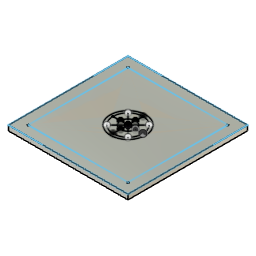
Rotator_Base_Mount_v9 (Autodesk Fusion 360 design; units mm, degrees)
Autodesk Fusion 360 part; units mm, degrees
sketch "Sketch1" plane through (0, 0, 0) normal (0, 0, 1) x (1, 0, 0)
  line L0 (-152.4, -152.4) -> (152.4, -152.4)
  line L1 (152.4, -152.4) -> (152.4, 152.4)
  line L2 (152.4, 152.4) -> (-152.4, 152.4)
  line L3 (-152.4, 152.4) -> (-152.4, -152.4)
  line L4 (-127, -127) -> (127, -127)
  line L5 (127, -127) -> (127, 127)
  line L6 (127, 127) -> (-127, 127)
  line L7 (-127, 127) -> (-127, -127)
  circle A0 centre (0, 0) radius 45
  circle A1 centre (0, 0) radius 38.1
  circle A2 centre (0, 0) radius 19.05
  line L8 (0, 0) -> (-38.1, 0)
  line L9 (0, 0) -> (0, 38.1)
  line L10 (0, 0) -> (38.1, 0)
  line L11 (0, 0) -> (0, -38.1)
  line L12 (0, 0) -> (26.9408, 26.9408)
  line L13 (0, 0) -> (38.1, 0) construction
  line L14 (0, 0) -> (26.9408, -26.9408)
  line L15 (0, 0) -> (38.1, 0) construction
  line L16 (0, 0) -> (-26.9408, -26.9408)
  line L17 (0, 0) -> (38.1, 0) construction
  line L18 (0, 0) -> (-26.9408, 26.9408)
  line L19 (0, 0) -> (38.1, 0) construction
  point P0 (0, 19.05)
  point P1 (19.05, 0)
  point P2 (0, -19.05)
  point P3 (-19.05, 0)
  dimension "d1" = 304.8
  dimension "d2" = 304.8
  dimension "d3" = 254
  dimension "d4" = 254
  dimension "d5" = 90
  dimension "d6" = 76.2
  dimension "d7" = 38.1
  dimension "d8" = 38.1
  dimension "d9" = 38.1
  dimension "d10" = 38.1
  dimension "d11" = 38.1
  dimension "d12" = 45
  dimension "d13" = 45
  dimension "d14" = 135
  dimension "d15" = 135
  constraint horizontal L0
  constraint vertical L1
  constraint horizontal L2
  constraint vertical L3
  constraint horizontal L4
  constraint vertical L5
  constraint horizontal L6
  constraint vertical L7
  constraint coincident A0.centre A1.centre
  constraint coincident A1 L8.end
  constraint horizontal L8
  constraint perpendicular L8 L9
  constraint parallel L8 L10
  constraint perpendicular L10 L11
  constraint horizontal L13
  constraint horizontal L15
  constraint horizontal L17
  constraint horizontal L19
  constraint midpoint L9 P0
  constraint midpoint L17 P1
  constraint midpoint L11 P2
  constraint midpoint L8 P3
  measures "d1" distance of L0.start L0.end
  measures "d2" distance of L0.start L2.end
  measures "d3" distance of L4.start L4.end
  measures "d4" distance of L4.start L6.end
  measures "d5" diameter of A0
  measures "d6" diameter of A1
  measures "d7" diameter of A2
  measures "d8" distance of A0.centre L8.end
  measures "d9" distance of A0.centre L9.end
  measures "d10" distance of A0.centre L10.end
  measures "d11" distance of A0.centre L11.end
  measures "d12" angle of L12 L13
  measures "d13" angle of L14 L15
  measures "d14" angle of L16 L17
  measures "d15" angle of L18 L19
extrude "Extrude1" add sketch "Sketch1" against normal blind 12.7 contours L0 L1 L2 L3 | L4 L5 L6 L7 | A0 | A1 A2 L10 L12 | A1 A2 L10 L14 | A1 A2 L9 L12 | A1 A2 L11 L14 | A2 L10 L12 | A2 L10 L14 | A1 A2 L9 L18 | A2 L9 L12 | A1 A2 L11 L16 | A2 L11 L14 | A2 L8 L16 | A2 L9 L18 | A2 L11 L16 | A2 L8 L18 | A1 A2 L8 L18 | A1 A2 L8 L16 makes body 1 in component "PT785S_Base_Mount"
hole "Hole1" at (-127, 127, 0) at (127, 127, 0) at (127, -127, 0) at (-127, -127, 0) at (-38.1, 0, 0) at (0, 38.1, 0) at (38.1, 0, 0) at (0, -38.1, 0) direction (0, 0, -1) diameter 5.1308 depth 12.7 tip angle 180 bodies 1 in component "PT785S_Base_Mount"
thread "Thread1" "ANSI Unified Screw Threads 0.25 1/4-20 UNC 1B" in component "PT785S_Base_Mount"
hole "Hole2" at (-26.9408, 26.9408, 0) at (26.9408, 26.9408, 0) at (26.9408, -26.9408, 0) at (-26.9408, -26.9408, 0) at (-19.05, 0, 0) at (0, 19.05, 0) at (19.05, 0, 0) at (0, -19.05, 0) direction (0, 0, -1) diameter 2.7686 depth 12.7 tip angle 180 bodies 1 in component "PT785S_Base_Mount"
thread "Thread2" "ANSI Unified Screw Threads 0.138(#6) 6-32 UNC 2B" in component "PT785S_Base_Mount"
hole "Hole3" at (0, 0, 0) direction (0, 0, -1) diameter 7.9756 depth 12.7 tip angle 180 bodies 1 in component "PT785S_Base_Mount"
thread "Thread3" "ANSI Unified Screw Threads 0.375 3/8-16 UNC 1B" in component "PT785S_Base_Mount"
copy_body "Body->Comp1" bodies 1 removing the originals makes body 2 in component "Aluminum_6061_Plate"
component "PT785S_Base_Mount" placed x (1, 0, 0) y (0, 1, 0) z (0, 0, 1) at (0, 0, 0)
component "Aluminum_6061_Plate" placed x (1, 0, 0) y (0, 1, 0) z (0, 0, 1) at (0, 0, 0) in component "PT785S_Base_Mount"
named bodies: "Aluminum_6061_Plate"
